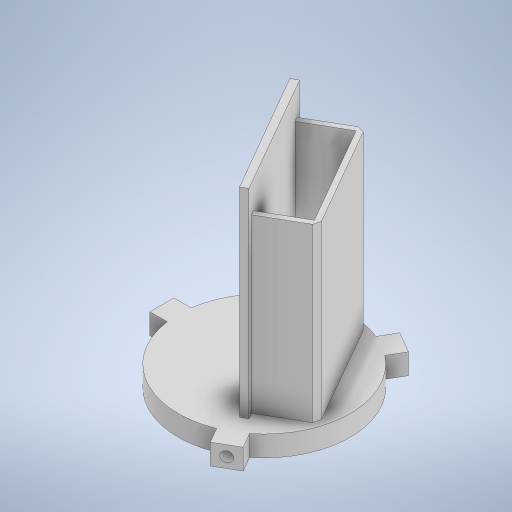
# Autodesk Inventor part: Electronic casing
Saved by Autodesk Inventor 2024 (Build 280153000, 153)
## iProperties
Created: 2024-03-27
Part Number: Electronic casing
Material: Generic
Document SubType Name: Modeling
Designer: auror
Density: 1 g/cm^3
Appearance: Default
Author: auror
Autodesk Inventor part; units mm, degrees
ref_plane "YZ Plane" through (0, 0, 0) normal (1, 0, 0) x (0, 1, 0)
ref_plane "XZ Plane" through (0, 0, 0) normal (0, 1, 0) x (-1, 0, 0)
ref_plane "XY Plane" through (0, 0, 0) normal (0, 0, 1) x (1, 0, 0)
sketch "Sketch9" plane through (0, 0, 0) normal (0, 1, 0) x (-1, 0, 0)
  line L0 (36.165, 0) -> (-40.8335, 0) construction
  line L1 (0, 0) -> (-26.8726, 46.5447) construction
  line L2 (0, 0) -> (-26.275, -45.5096) construction
  line L3 (29.7951, 3.5) -> (29.7951, -3.5)
  line L4 (29.7951, 3.5) -> (24.7538, 3.5)
  line L5 (29.7951, -3.5) -> (24.7538, -3.5)
  line L6 (0, 0) -> (-18.4784, 42.9064) construction
  line L7 (0, 0) -> (-25.1787, 33.7798) construction
  line L8 (0, 0) -> (29.7951, 3.5) construction
  line L9 (-11.8664, 27.5534) -> (-17.9288, 24.0533)
  line L10 (-11.8664, 27.5534) -> (-9.3457, 23.1875)
  line L11 (-17.9288, 24.0533) -> (-15.4081, 19.6873)
  line L12 (0, 0) -> (-18.2948, -42.48) construction
  line L13 (-18.2948, -42.48) -> (0, 0) construction
  line L14 (0, 0) -> (-26.6993, -35.8199) construction
  line L15 (-17.9288, -24.0533) -> (-11.8664, -27.5534)
  line L16 (-17.9288, -24.0533) -> (-15.4081, -19.6873)
  line L17 (-11.8664, -27.5534) -> (-9.3457, -23.1875)
  arc A0 (-15.4081, 19.6873) -> (-15.4081, -19.6873) centre (0, 0) ccw
  arc A1 (-9.3457, -23.1875) -> (24.7538, -3.5) centre (0, 0) ccw
  arc A2 (24.7538, 3.5) -> (-9.3457, 23.1875) centre (0, 0) ccw
  dimension "d131" = 120
  dimension "d132" = 120
  dimension "d133" = 7
  dimension "d134" = 3.5
  dimension "d136" = 6.7
  dimension "d137" = 6.7
  dimension "d138" = 6.7
  dimension "d139" = 6.7
  dimension "d140" = 6.7
  constraints: 36 end point, 6 point on circle, 4 perpendicular, 4 point on line, 3 centre point, 3 horizontal, 2 coincident, 1 vertical
  measures "d131" angle of L2 L0
  measures "d132" angle of L1 L0
  measures "d133" distance of L3.end L3.start
  measures "d134" distance from line of L0 L3.start
  measures "d136" angle of L1 L6
  measures "d137" angle of L7 L1
  measures "d138" angle of L0 L8
  measures "d139" angle of L2 L12
  measures "d140" angle of L2 L14
extrude "Extrusion4" add sketch "Sketch9" along normal blind 6
sketch "Sketch10" plane through (17.9288, 0, 24.0533) normal (0.5, 0, 0.8660254) x (0.8660254, 0, -0.5)
  line L0 (0, 0) -> (0, 6) projected
  line L1 (-7.0002, 0) -> (0, 0) projected
  point P0 (-3.5001, 0)
  point P1 (-3.5, 3)
  point P2 (0, 3)
  dimension "d143" = 3.5
  dimension "d144" = 3
  constraints: 1 midpoint
  measures "d143" distance of point (0, 3) point (-3.5, 3)
  measures "d144" distance from line of L1 point (-3.5, 3)
hole "Hole5" at (14.8977, 3, 25.8033) direction (-0.5, 0, -0.8660254) diameter 3 depth 15 tip angle 118 counterbore diameter 4 counterbore depth 0
sketch "Sketch11" plane through (11.8664, 0, -27.5534) normal (0.5, 0, -0.8660254) x (-0.8660254, 0, -0.5)
  line L0 (-7.0002, 0) -> (0, 0) projected
  point P0 (-3.5001, 0)
  point P1 (-3.5001, 3)
  dimension "d152" = 3
  measures "d152" distance from line of L0 point (-3.5, 3)
hole "Hole6" at (14.8976, 3, -25.8033) direction (-0.5, 0, 0.8660254) diameter 3 depth 15 tip angle 118 counterbore diameter 4 counterbore depth 0
sketch "Sketch12" plane through (-29.7951, 0, -3.5) normal (-1, 0, 0) x (0, 0, 1)
  line L0 (0, 0) -> (7, 0) projected
  point P0 (3.5, 0)
  point P1 (3.5, 3)
  dimension "d160" = 3
  measures "d160" distance from line of L0 point (3.5, 3)
hole "Hole7" at (-29.7951, 3, 0) direction (1, 0, 0) diameter 3 depth 15 tip angle 118 counterbore diameter 4 counterbore depth 0
sketch "Sketch13" plane through (0, 6, 0) normal (0, 1, 0) x (1, 0, 0)
  line L0 (0, -31.2314) -> (0, 39.2316) construction
  line L1 (12.2945, -21.2947) -> (-12.5, 21.6506) construction
  arc A0 (9.3457, 23.1875) -> (-24.7538, 3.5) centre (0, 0) ccw construction
  line L2 (9.82, -17.0087) -> (11.552, -16.0087)
  line L3 (9.82, -17.0087) -> (-10.18, 17.6324)
  line L4 (-10.18, 17.6324) -> (-8.3869, 18.6676)
  line L5 (-8.3869, 18.6676) -> (11.552, -16.0087)
  dimension "d168" = -30
  dimension "d169" = 0
  dimension "d176" = 40
  dimension "d178" = 2
  constraints: 12 end point, 2 perpendicular, 2 point on line, 1 collinear, 1 point on circle, 1 vertical
  measures "d168" angle of L0 L1
  measures "d169" distance from line of A0.centre L1
  measures "d176" distance of L3.end L2.start
  measures "d178" distance of L2.start L2.end
extrude "Extrusion5" add sketch "Sketch13" along normal blind 58
sketch "Sketch14" plane through (0, 6, 0) normal (0, 1, 0) x (1, 0, 0)
  line L0 (11.552, -16.0087) -> (-8.3869, 18.6676) projected
  line L1 (-8.3869, 18.6676) -> (11.552, -16.0087) projected
  line L2 (1.5826, 1.3295) -> (16.735, 10.0421) construction
  line L3 (21.0771, -6.4944) -> (4.6276, 22.1135)
  line L4 (4.6276, 22.1135) -> (-6.6422, 15.6334)
  line L5 (21.0771, -6.4944) -> (9.8074, -12.9745)
  line L6 (3.8799, 23.4139) -> (23.6749, -11.0122) construction
  line L7 (9.8074, -12.9745) -> (26.3984, -3.4346) construction
  line L8 (-6.6422, 15.6334) -> (9.3457, 24.8265) construction
  line L9 (21.8248, -7.7947) -> (10.5551, -14.2749)
  line L10 (3.8799, 23.4139) -> (-7.3899, 16.9338)
  line L11 (22.3775, -5.7467) -> (5.9279, 22.8612)
  line L12 (3.8799, 23.4139) -> (5.9279, 22.8612)
  line L13 (22.3775, -5.7467) -> (21.8248, -7.7947)
  point P0 (0, 0)
  point P1 (-6.6422, 15.6334)
  dimension "d181" = 13
  dimension "d182" = 13
  dimension "d184" = 20
  dimension "d185" = 16.5
  dimension "d186" = 33
  dimension "d192" = 1.5
  dimension "d193" = 1.5
  dimension "d194" = 1.5
  dimension "d195" = 1.5
  constraints: 24 end point, 10 point on line, 6 perpendicular, 2 coincident, 1 parallel
  measures "d181" distance from line of L0 L3.start
  measures "d182" distance from line of L0 L3.end
  measures "d184" distance of point (11.552, -16.009) L2.start
  measures "d185" distance from line of L2 L3.start
  measures "d186" distance of L3.end L3.start
  measures "d192" distance of L3.start L9.start
  measures "d193" distance of L6.start L3.end
  measures "d194" distance of L3.start L11.start
  measures "d195" distance of L3.end L11.end
extrude "Extrusion6" add sketch "Sketch14" along normal blind 50 contours L0 L5 L3 L4 L10 L12 L11 L13 L9
body "Solid2"
